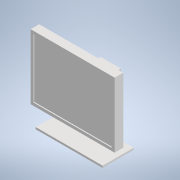
# Autodesk Inventor part: Monitor
Saved by Autodesk Inventor 2022 (Build 260153000, 153)
## iProperties
Created: 2023-12-20
Part Number: Monitor
Material: Generic
Document SubType Name: Modeling
Designer: Petr Černý
Density: 1 g/cm^3
Appearance: Default
Author: Petr Černý
Autodesk Inventor part; units mm, degrees
ref_plane "YZ Plane" through (0, 0, 0) normal (1, 0, 0) x (0, 1, 0)
ref_plane "XZ Plane" through (0, 0, 0) normal (0, 1, 0) x (-1, 0, 0)
ref_plane "XY Plane" through (0, 0, 0) normal (0, 0, 1) x (1, 0, 0)
sketch "Sketch1" plane through (0, 0, 0) normal (0, 0, 1) x (1, 0, 0)
  line L0 (90.3787, -90.3787) -> (-349.6213, -90.3787)
  line L1 (-349.6213, -90.3787) -> (-349.6213, -430.3787)
  line L2 (-349.6213, -430.3787) -> (90.3787, -430.3787)
  line L3 (90.3787, -430.3787) -> (90.3787, -90.3787)
  point P0 (0, 0)
  dimension "d0" = 440
  dimension "d1" = 340
  constraints: 8 end point, 2 parallel, 1 horizontal, 1 perpendicular
  measures "d0" distance of L2.end L1.end
  measures "d1" distance of L1.end L0.end
extrude "Extrusion1" add sketch "Sketch1" along normal blind 45
sketch "Sketch2" plane through (0, 0, 45) normal (0, 0, 1) x (1, 0, 0)
  line L0 (-334.6213, -105.3787) -> (75.3787, -105.3787)
  line L1 (75.3787, -105.3787) -> (75.3787, -415.3787)
  line L2 (75.3787, -415.3787) -> (-334.6213, -415.3787)
  line L3 (-334.6213, -415.3787) -> (-334.6213, -105.3787)
  line L4 (90.3787, -430.3787) -> (90.3787, -90.3787) projected
  line L5 (90.3787, -90.3787) -> (-349.6213, -90.3787) projected
  point P0 (0, 0)
  dimension "d4" = 410
  dimension "d5" = 310
  dimension "d6" = 15
  dimension "d7" = 15
  constraints: 8 end point, 2 parallel, 1 horizontal, 1 perpendicular
  measures "d4" distance of L0.start L0.end
  measures "d5" distance of L0.end L1.end
  measures "d6" distance between parallel lines of L4 L1
  measures "d7" distance between parallel lines of L5 L0
extrude "Extrusion2" cut sketch "Sketch2" against normal blind 5
sketch "Sketch3" plane through (0, 0, 0) normal (0, 0, -1) x (-1, 0, 0)
  line L0 (-35.3787, -145.3787) -> (294.6213, -145.3787)
  line L1 (294.6213, -145.3787) -> (294.6213, -375.3787)
  line L2 (294.6213, -375.3787) -> (-35.3787, -375.3787)
  line L3 (-35.3787, -375.3787) -> (-35.3787, -145.3787)
  line L4 (349.6213, -430.3787) -> (-90.3787, -430.3787) projected
  line L5 (-90.3787, -430.3787) -> (-90.3787, -90.3787) projected
  point P0 (0, 0)
  dimension "d10" = 330
  dimension "d11" = 230
  dimension "d12" = 55
  dimension "d13" = 55
  constraints: 8 end point, 2 parallel, 1 horizontal, 1 perpendicular
  measures "d10" distance of L1.end L2.end
  measures "d11" distance of L0.end L1.end
  measures "d12" distance between parallel lines of L4 L2
  measures "d13" distance between parallel lines of L5 L3
extrude "Extrusion3" add sketch "Sketch3" along normal blind 42
sketch "Sketch4" plane through (0, 0, -42) normal (0, 0, -1) x (-1, 0, 0)
  line L0 (-35.3787, -375.3787) -> (294.6213, -375.3787) projected
  line L1 (294.6213, -375.3787) -> (294.6213, -145.3787) projected
  line L2 (294.6213, -145.3787) -> (-35.3787, -145.3787) projected
  line L3 (-35.3787, -145.3787) -> (-35.3787, -375.3787) projected
  line L4 (77.1213, -232.8787) -> (182.1213, -232.8787)
  line L5 (182.1213, -232.8787) -> (182.1213, -287.8787)
  line L6 (182.1213, -287.8787) -> (77.1213, -287.8787)
  line L7 (77.1213, -287.8787) -> (77.1213, -232.8787)
  point P0 (0, 0)
  dimension "d16" = 105
  dimension "d17" = 55
  dimension "d18" = 87.5
  dimension "d19" = 112.5
  constraints: 8 end point, 2 parallel, 1 horizontal, 1 perpendicular
  measures "d16" distance of L5.end L6.end
  measures "d17" distance of L4.end L5.end
  measures "d18" distance between parallel lines of L2 L4
  measures "d19" distance between parallel lines of L3 L7
extrude "Extrusion4" add sketch "Sketch4" along normal blind 58 contours L4 L5 L6 L7
sketch "Sketch5" plane through (-182.1213, -232.8787, -42) normal (0, 1, 0) x (1, 0, 0)
  line L0 (105, 58) -> (0, 58) projected
  line L1 (105, 58) -> (0, 58)
  line L2 (0, 58) -> (0, 113)
  line L3 (0, 113) -> (105, 113)
  line L4 (105, 113) -> (105, 58)
  point P0 (182.1213, -42)
  dimension "d22" = 105
  dimension "d23" = 55
  constraints: 8 end point, 2 parallel, 1 horizontal, 1 perpendicular
  measures "d22" distance of L2.end L3.end
  measures "d23" distance of L1.end L2.end
extrude "Extrusion5" add sketch "Sketch5" against normal blind 280
sketch "Sketch6" plane through (-182.1213, -512.8787, -42) normal (0, -1, 0) x (1, 0, 0)
  line L0 (0, -113) -> (105, -113) projected
  line L1 (105, -113) -> (105, -58) projected
  line L2 (105, -58) -> (0, -58) projected
  line L3 (0, -58) -> (0, -113) projected
  line L4 (227.5, -58) -> (-122.5, -58)
  line L5 (-122.5, -58) -> (-122.5, 105)
  line L6 (-122.5, 105) -> (227.5, 105)
  line L7 (227.5, 105) -> (227.5, -58)
  line L8 (-167.5, 42) -> (-167.5, 87) projected
  point P0 (182.1213, 42)
  dimension "d26" = 350
  dimension "d27" = 163
  dimension "d28" = 0
  dimension "d29" = 45
  constraints: 8 end point, 2 parallel, 1 horizontal, 1 perpendicular
  measures "d26" distance of L5.end L6.end
  measures "d27" distance of L4.end L5.end
  measures "d28" distance between parallel lines of L2 L4
  measures "d29" distance between parallel lines of L8 L5
extrude "Extrusion6" add sketch "Sketch6" against normal blind 10 contours L4 L5 L6 L7 L2
body "Solid1"
